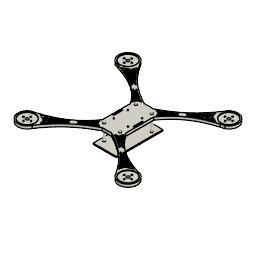
drone_frame_design (Autodesk Fusion 360 design; units mm, degrees)
part number: 2026-03-04-22-05-30-205
Autodesk Fusion 360 part; units mm, degrees
(part 1 of 3)
sketch "Sketch1" plane through (0, 0, 0) normal (0, 0, 1) x (1, 0, 0)
  line L0 (10, -45) -> (-10, -45)
  line L1 (-25, -30) -> (-25, 30)
  line L2 (-10, 45) -> (10, 45)
  line L3 (25, 30) -> (25, -30)
  line L4 (10, 45) -> (25, 30)
  line L5 (-25, 30) -> (-10, 45)
  line L6 (-10, -45) -> (-25, -30)
  line L7 (10, -45) -> (25, -30)
  circle A0 centre (108, 108) radius 20
  line L8 (0, 2.5) -> (0, 20)
  circle A1 centre (-108, 108) radius 20
  line L9 (20, 0) -> (2.5, 0)
  circle A2 centre (-108, -108) radius 20
  circle A3 centre (108, -108) radius 20
  line L10 (10, 45) -> (0, 45)
  spline S0 degree 5 poles (10, 45) (11.9791, 46.0284) (15.9034, 48.1188) (21.6887, 51.3552) (29.1964, 55.8754) (38.2146, 61.8908) (46.833, 68.3041) (55.0184, 75.1487) (62.7516, 82.4437) (70.0489, 90.1727) (76.9426, 98.3036) (82.1609, 105.1037) (85.9183, 110.3595) (88.3548, 113.9314) (89.5561, 115.7344) knots 0 0 0 0 0 0 0.1 0.2 0.3 0.4 0.5 0.6 0.7 0.8 0.9 1 1 1 1 1 1
  spline S1 degree 5 poles (25, 30) (26.2769, 31.7834) (28.8813, 35.2989) (32.9395, 40.4185) (38.6588, 46.9323) (46.356, 54.5193) (54.6474, 61.5042) (63.577, 67.8424) (73.161, 73.5176) (83.3647, 78.5649) (94.1376, 83.0355) (103.1721, 86.1903) (110.1669, 88.3346) (114.9258, 89.6671) (117.3292, 90.3092) knots 0 0 0 0 0 0 0.1 0.2 0.3 0.4 0.5 0.6 0.7 0.8 0.9 1 1 1 1 1 1
  spline S2 degree 5 poles (-10, 45) (-11.9791, 46.0284) (-15.9034, 48.1188) (-21.6887, 51.3552) (-29.1964, 55.8754) (-38.2146, 61.8908) (-46.833, 68.3041) (-55.0184, 75.1487) (-62.7516, 82.4437) (-70.0489, 90.1727) (-76.9426, 98.3036) (-82.1609, 105.1037) (-85.9183, 110.3595) (-88.3548, 113.9314) (-89.5561, 115.7344) knots 0 0 0 0 0 0 0.1 0.2 0.3 0.4 0.5 0.6 0.7 0.8 0.9 1 1 1 1 1 1
  line L11 (-0.5595, 39.5129) -> (20.5595, 50.4871)
  line L12 (83.0456, 105.9625) -> (96.0665, 125.5063)
  line L13 (0.5595, 39.5129) -> (-20.5595, 50.4871)
  line L14 (-83.0456, 105.9625) -> (-96.0665, 125.5063)
  spline S3 degree 5 poles (-25, 30) (-26.2769, 31.7834) (-28.8813, 35.2989) (-32.9395, 40.4185) (-38.6588, 46.9323) (-46.356, 54.5193) (-54.6474, 61.5042) (-63.577, 67.8424) (-73.161, 73.5176) (-83.3647, 78.5649) (-94.1376, 83.0355) (-103.1721, 86.1903) (-110.1669, 88.3346) (-114.9258, 89.6671) (-117.3292, 90.3092) knots 0 0 0 0 0 0 0.1 0.2 0.3 0.4 0.5 0.6 0.7 0.8 0.9 1 1 1 1 1 1
  line L15 (17.8241, 19.9779) -> (32.1759, 40.0221)
  line L16 (104.7277, 86.9428) -> (129.9307, 93.6755)
  line L17 (-17.8241, 19.9779) -> (-32.1759, 40.0221)
  line L18 (-104.7277, 86.9428) -> (-129.9307, 93.6755)
  spline S4 degree 5 poles (-25, -30) (-26.2769, -31.7834) (-28.8813, -35.2989) (-32.9395, -40.4185) (-38.6588, -46.9323) (-46.356, -54.5193) (-54.6474, -61.5042) (-63.577, -67.8424) (-73.161, -73.5176) (-83.3647, -78.5649) (-94.1376, -83.0355) (-103.1721, -86.1903) (-110.1669, -88.3346) (-114.9258, -89.6671) (-117.3292, -90.3092) knots 0 0 0 0 0 0 0.1 0.2 0.3 0.4 0.5 0.6 0.7 0.8 0.9 1 1 1 1 1 1
  line L19 (-17.8241, -19.9779) -> (-32.1759, -40.0221)
  line L20 (-104.7277, -86.9428) -> (-129.9307, -93.6755)
  spline S5 degree 5 poles (-10, -45) (-11.9791, -46.0284) (-15.9034, -48.1188) (-21.6887, -51.3552) (-29.1964, -55.8754) (-38.2146, -61.8908) (-46.833, -68.3041) (-55.0184, -75.1487) (-62.7516, -82.4437) (-70.0489, -90.1727) (-76.9426, -98.3036) (-82.1609, -105.1037) (-85.9183, -110.3595) (-88.3548, -113.9314) (-89.5561, -115.7344) knots 0 0 0 0 0 0 0.1 0.2 0.3 0.4 0.5 0.6 0.7 0.8 0.9 1 1 1 1 1 1
  line L21 (0.5595, -39.5129) -> (-20.5595, -50.4871)
  line L22 (-83.0456, -105.9625) -> (-96.0665, -125.5063)
  spline S6 degree 5 poles (10, -45) (11.9791, -46.0284) (15.9034, -48.1188) (21.6887, -51.3552) (29.1964, -55.8754) (38.2146, -61.8908) (46.833, -68.3041) (55.0184, -75.1487) (62.7516, -82.4437) (70.0489, -90.1727) (76.9426, -98.3036) (82.1609, -105.1037) (85.9183, -110.3595) (88.3548, -113.9314) (89.5561, -115.7344) knots 0 0 0 0 0 0 0.1 0.2 0.3 0.4 0.5 0.6 0.7 0.8 0.9 1 1 1 1 1 1
  line L23 (-0.5595, -39.5129) -> (20.5595, -50.4871)
  line L24 (83.0456, -105.9625) -> (96.0665, -125.5063)
  spline S7 degree 5 poles (25, -30) (26.2769, -31.7834) (28.8813, -35.2989) (32.9395, -40.4185) (38.6588, -46.9323) (46.356, -54.5193) (54.6474, -61.5042) (63.577, -67.8424) (73.161, -73.5176) (83.3647, -78.5649) (94.1376, -83.0355) (103.1721, -86.1903) (110.1669, -88.3346) (114.9258, -89.6671) (117.3292, -90.3092) knots 0 0 0 0 0 0 0.1 0.2 0.3 0.4 0.5 0.6 0.7 0.8 0.9 1 1 1 1 1 1
  line L25 (17.8241, -19.9779) -> (32.1759, -40.0221)
  line L26 (104.7277, -86.9428) -> (129.9307, -93.6755)
  line L27 (20, 0) -> (2.5, 0)
  line L28 (-128, 128) -> (-128, 108)
  line L29 (-128, -108) -> (-128, -128)
  line L30 (128, 128) -> (108, 128)
  line L31 (-108, 128) -> (-128, 128)
  line L32 (128, -128) -> (128, -108)
  line L33 (128, 108) -> (128, 128)
  line L34 (-128, -128) -> (-108, -128)
  line L35 (108, -128) -> (128, -128)
  point P0 (25, -45)
  point P1 (-25, -45)
  point P2 (-25, 45)
  point P3 (25, 45)
  point P4 (55.2098, 75.5318)
  point P5 (62.16, 66.6356)
  point P6 (-55.2098, 75.5318)
  point P7 (-62.16, 66.6356)
  point P8 (-62.16, -66.6356)
  point P9 (-55.2098, -75.5318)
  point P10 (55.2098, -75.5318)
  point P11 (62.16, -66.6356)
  dimension "d1" = 256
  dimension "d2" = 256
  dimension "d3" = 50
  dimension "d4" = 90
  dimension "d7" = 15
  dimension "d8" = 15
  dimension "d9" = 15
  dimension "d10" = 15
  dimension "d11" = 15
  dimension "d12" = 15
  dimension "d13" = 15
  dimension "d14" = 15
  dimension "d15" = 40
  constraint horizontal L30
  constraint perpendicular L28 L31
  constraint parallel L30 L35
  constraint parallel L28 L33
  constraint horizontal L0
  constraint perpendicular L0 L1
  constraint parallel L0 L2
  constraint parallel L1 L3
  constraint coincident P3 L2
  constraint coincident P3 L3
  constraint coincident P2 L1
  constraint coincident P2 L2
  constraint coincident P1 L0
  constraint coincident P1 L1
  constraint coincident P0 L0
  constraint coincident P0 L3
  constraint tangent A0 L30
  constraint tangent A0 L33
  constraint symmetric A0 L8 A1
  constraint symmetric A0 L9 A3
  constraint symmetric A1 L9 A2
  constraint midpoint L2 L10.end
  constraint symmetric L1 L3 L8
  constraint symmetric L0 L2 L9
  constraint coincident A0 S0.end
  constraint coincident A0 S1.end
  constraint midpoint L2.end L11
  constraint midpoint S0.end L12
  constraint midpoint L3.start L15
  constraint midpoint S1.end L16
  constraint symmetric L2.end L8 L2.start
  constraint symmetric L3.start L8 L1.end
  constraint symmetric L8 P4 P6
  constraint symmetric L8 S0.end S2.end
  constraint symmetric L8 P5 P7
  constraint symmetric L8 S1.end S3.end
  constraint symmetric L8 L11.start L13.start
  constraint symmetric L8 L11.end L13.end
  constraint symmetric L8 L12.start L14.start
  constraint symmetric L8 L12.end L14.end
  constraint symmetric L8 L15.start L17.start
  constraint symmetric L8 L15.end L17.end
  constraint symmetric L8 L16.start L18.start
  constraint symmetric L8 L16.end L18.end
  constraint symmetric L2.end L9 L0.start
  constraint symmetric L3.start L9 L3.end
  constraint symmetric L27.start L9 L9.start
  constraint symmetric L27.end L9 L9.end
  constraint symmetric L9 P4 P10
  constraint symmetric L9 S0.end S6.end
  constraint symmetric L9 P5 P11
  constraint symmetric L9 S1.end S7.end
  constraint symmetric L9 L2.start L0.end
  constraint symmetric L9 P6 P9
  constraint symmetric L9 S2.end S5.end
  constraint symmetric L9 L11.start L23.start
  constraint symmetric L9 L11.end L23.end
  constraint symmetric L9 L12.start L24.start
  constraint symmetric L9 L12.end L24.end
  constraint symmetric L9 L13.start L21.start
  constraint symmetric L9 L13.end L21.end
  constraint symmetric L9 L14.start L22.start
  constraint symmetric L9 L14.end L22.end
  constraint symmetric L9 L1.end L1.start
  constraint symmetric L9 P7 P8
  constraint symmetric L9 S3.end S4.end
  constraint symmetric L9 L15.start L25.start
  constraint symmetric L9 L15.end L25.end
  constraint symmetric L9 L16.start L26.start
  constraint symmetric L9 L16.end L26.end
  constraint symmetric L9 L17.start L19.start
  constraint symmetric L9 L17.end L19.end
  constraint symmetric L9 L18.start L20.start
  constraint symmetric L9 L18.end L20.end
  constraint coincident A1 L28.end
  constraint coincident A2 L29.start
  constraint collinear L28 L29
  constraint coincident A0 L30.end
  constraint coincident A1 L31.start
  constraint collinear L30 L31
  constraint coincident A3 L32.end
  constraint coincident A0 L33.start
  constraint collinear L32 L33
  constraint coincident A2 L34.end
  constraint coincident A3 L35.start
  constraint collinear L34 L35
  measures "d1" distance of L29.end L32.start
  measures "d2" distance of L28.start L29.end
  measures "d3" distance of P2 P3
  measures "d4" distance of P1 P2
  measures "d7" distance of P3 L2.end L29.end
  measures "d8" distance of P3 L3.start L29.end
  measures "d9" distance of P2 L1.end
  measures "d10" distance of P2 L2.start
  measures "d11" distance of P1 L0.end
  measures "d12" distance of P1 L1.start
  measures "d13" distance of P0 L0.start
  measures "d14" distance of P0 L3.end
  measures "d15" diameter of A0
sketch "Sketch3" plane through (0, 0, 0) normal (0, 0, 1) x (1, 0, 0)
extrude "Extrude1" add sketch "Sketch1" along normal blind 6 contours L1 L3 L4 L5 L6 L7 L11 L13 L21 L23 | L0 L21 L23 | L2 L10 L11 L13 makes body 1
extrude "Extrude2" add sketch "Sketch1" along normal blind 6 contours L7 A3 S6 S7 | L6 A2 S4 S5 | L4 A0 S0 S1 | L5 A1 S2 S3 bodies 1
sketch "Sketch4" plane through (0, 0, 6) normal (0, 0, 1) x (-1, 0, 0)
  spline S0 degree 5 poles (-10, 45) (-11.9791, 46.0284) (-15.9034, 48.1188) (-21.6887, 51.3552) (-29.1964, 55.8754) (-38.2146, 61.8908) (-46.833, 68.3041) (-55.0184, 75.1487) (-62.7516, 82.4437) (-70.0489, 90.1727) (-76.9426, 98.3036) (-82.1609, 105.1037) (-85.9183, 110.3595) (-88.3548, 113.9314) (-89.5561, 115.7344) knots 0 0 0 0 0 0 0.1 0.2 0.3 0.4 0.5 0.6 0.7 0.8 0.9 1 1 1 1 1 1
  arc A0 (-109.3801, 88.0477) -> (-89.5561, 115.7344) centre (-108, 108) ccw
  spline S1 degree 5 poles (-109.3801, 88.0477) (-108.6093, 87.8146) (-105.5101, 86.8635) (-100.1552, 85.1208) (-92.6931, 82.436) (-83.3647, 78.5649) (-73.161, 73.5176) (-63.577, 67.8424) (-54.6474, 61.5042) (-46.356, 54.5193) (-38.6588, 46.9323) (-32.9395, 40.4185) (-28.8813, 35.2989) (-26.2769, 31.7834) (-25, 30) knots -0.932954 -0.932954 -0.932954 -0.932954 -0.932954 -0.932954 -0.9 -0.8 -0.7 -0.6 -0.5 -0.4 -0.3 -0.2 -0.1 0 0 0 0 0 0
  line L0 (-10, 45) -> (-25, 30)
  line L1 (-10, -45) -> (10, -45)
  spline S2 degree 5 poles (10, -45) (11.9791, -46.0284) (15.9034, -48.1188) (21.6887, -51.3552) (29.1964, -55.8754) (38.2146, -61.8908) (46.833, -68.3041) (55.0184, -75.1487) (62.7516, -82.4437) (70.0489, -90.1727) (76.9426, -98.3036) (82.1609, -105.1037) (85.9183, -110.3595) (88.3548, -113.9314) (89.5561, -115.7344) knots 0 0 0 0 0 0 0.1 0.2 0.3 0.4 0.5 0.6 0.7 0.8 0.9 1 1 1 1 1 1
  arc A1 (109.3801, -88.0477) -> (89.5561, -115.7344) centre (108, -108) ccw
  spline S3 degree 5 poles (109.3801, -88.0477) (108.6093, -87.8146) (105.5101, -86.8635) (100.1552, -85.1208) (92.6931, -82.436) (83.3647, -78.5649) (73.161, -73.5176) (63.577, -67.8424) (54.6474, -61.5042) (46.356, -54.5193) (38.6588, -46.9323) (32.9395, -40.4185) (28.8813, -35.2989) (26.2769, -31.7834) (25, -30) knots -0.932954 -0.932954 -0.932954 -0.932954 -0.932954 -0.932954 -0.9 -0.8 -0.7 -0.6 -0.5 -0.4 -0.3 -0.2 -0.1 0 0 0 0 0 0
  line L2 (25, -30) -> (25, 30)
  spline S4 degree 5 poles (25, 30) (26.2769, 31.7834) (28.8813, 35.2989) (32.9395, 40.4185) (38.6588, 46.9323) (46.356, 54.5193) (54.6474, 61.5042) (63.577, 67.8424) (73.161, 73.5176) (83.3647, 78.5649) (92.6931, 82.436) (100.1552, 85.1208) (105.5101, 86.8635) (108.6093, 87.8146) (109.3801, 88.0477) knots 0 0 0 0 0 0 0.1 0.2 0.3 0.4 0.5 0.6 0.7 0.8 0.9 0.932954 0.932954 0.932954 0.932954 0.932954 0.932954
  arc A2 (89.5561, 115.7344) -> (109.3801, 88.0477) centre (108, 108) ccw
  spline S5 degree 5 poles (89.5561, 115.7344) (88.3548, 113.9314) (85.9183, 110.3595) (82.1609, 105.1037) (76.9426, 98.3036) (70.0489, 90.1727) (62.7516, 82.4437) (55.0184, 75.1487) (46.833, 68.3041) (38.2146, 61.8908) (29.1964, 55.8754) (21.6887, 51.3552) (15.9034, 48.1188) (11.9791, 46.0284) (10, 45) knots -1 -1 -1 -1 -1 -1 -0.9 -0.8 -0.7 -0.6 -0.5 -0.4 -0.3 -0.2 -0.1 0 0 0 0 0 0
  line L3 (10, 45) -> (-10, 45)
  line L4 (-25, 30) -> (-25, -30)
  spline S6 degree 5 poles (-25, -30) (-26.2769, -31.7834) (-28.8813, -35.2989) (-32.9395, -40.4185) (-38.6588, -46.9323) (-46.356, -54.5193) (-54.6474, -61.5042) (-63.577, -67.8424) (-73.161, -73.5176) (-83.3647, -78.5649) (-92.6931, -82.436) (-100.1552, -85.1208) (-105.5101, -86.8635) (-108.6093, -87.8146) (-109.3801, -88.0477) knots 0 0 0 0 0 0 0.1 0.2 0.3 0.4 0.5 0.6 0.7 0.8 0.9 0.932954 0.932954 0.932954 0.932954 0.932954 0.932954
  arc A3 (-89.5561, -115.7344) -> (-109.3801, -88.0477) centre (-108, -108) ccw
  spline S7 degree 5 poles (-89.5561, -115.7344) (-88.3548, -113.9314) (-85.9183, -110.3595) (-82.1609, -105.1037) (-76.9426, -98.3036) (-70.0489, -90.1727) (-62.7516, -82.4437) (-55.0184, -75.1487) (-46.833, -68.3041) (-38.2146, -61.8908) (-29.1964, -55.8754) (-21.6887, -51.3552) (-15.9034, -48.1188) (-11.9791, -46.0284) (-10, -45) knots -1 -1 -1 -1 -1 -1 -0.9 -0.8 -0.7 -0.6 -0.5 -0.4 -0.3 -0.2 -0.1 0 0 0 0 0 0
sketch "Sketch5" plane through (0, 0, 6) normal (0, 0, 1) x (-1, 0, 0)
  spline S0 degree 5 poles (-25, -30) (-26.2769, -31.7834) (-28.8813, -35.2989) (-32.9395, -40.4185) (-38.6588, -46.9323) (-46.356, -54.5193) (-54.6474, -61.5042) (-63.577, -67.8424) (-73.161, -73.5176) (-83.3647, -78.5649) (-92.6931, -82.436) (-100.1552, -85.1208) (-105.5101, -86.8635) (-108.6093, -87.8146) (-109.3801, -88.0477) knots 0 0 0 0 0 0 0.1 0.2 0.3 0.4 0.5 0.6 0.7 0.8 0.9 0.932954 0.932954 0.932954 0.932954 0.932954 0.932954
  arc A0 (-89.5561, -115.7344) -> (-109.3801, -88.0477) centre (-108, -108) ccw
  spline S1 degree 5 poles (-89.5561, -115.7344) (-88.3548, -113.9314) (-85.9183, -110.3595) (-82.1609, -105.1037) (-76.9426, -98.3036) (-70.0489, -90.1727) (-62.7516, -82.4437) (-55.0184, -75.1487) (-46.833, -68.3041) (-38.2146, -61.8908) (-29.1964, -55.8754) (-21.6887, -51.3552) (-15.9034, -48.1188) (-11.9791, -46.0284) (-10, -45) knots -1 -1 -1 -1 -1 -1 -0.9 -0.8 -0.7 -0.6 -0.5 -0.4 -0.3 -0.2 -0.1 0 0 0 0 0 0
  line L0 (-16.6491, -44.0078) -> (-24.5394, -36.1175)
  line L1 (-16.6491, -44.0078) -> (-15.7266, -44.9303)
  line L2 (-24.5394, -36.1175) -> (-26.1093, -34.5476)
  spline S2 degree 3 poles (-86.4629, -107.5181) (-77.6632, -95.0692) (-67.8257, -83.6168) (-56.6007, -73.5039) (-44.7534, -62.8301) (-31.3991, -53.6699) (-16.9588, -45.6135) (-16.549, -45.3849) (-16.1382, -45.1571) (-15.7266, -44.9303) knots -0.921557 -0.921557 -0.921557 -0.921557 -0.5 -0.5 -0.5 -0.055069 -0.055069 -0.055069 -0.042441 -0.042441 -0.042441 -0.042441
  spline S3 degree 3 poles (-26.1093, -34.5476) (-33.7424, -44.66) (-42.377, -53.7768) (-52.2721, -61.6437) (-60.5587, -68.2317) (-69.767, -73.8901) (-79.7914, -78.6767) (-86.5715, -81.9141) (-93.7109, -84.7689) (-101.1598, -87.3016) knots 0.039267 0.039267 0.039267 0.039267 0.383484 0.383484 0.383484 0.671746 0.671746 0.671746 0.86671 0.86671 0.86671 0.86671
  circle A1 centre (-108, -108) radius 20
  line L3 (-21.0824, -39.4285) -> (-91.6554, -96.5652)
  line L4 (-19.9851, -40.7292) -> (-90.7737, -97.8385)
  line L5 (-15.7266, -44.9303) -> (-22.1293, -42.4591)
  line L6 (-22.1293, -42.4591) -> (-21.2525, -48.0608)
  line L7 (-23.5672, -43.6191) -> (-22.7358, -48.9312)
  line L8 (-18.5197, -42.1372) -> (-20.6913, -41.299)
  line L9 (-22.7358, -48.9312) -> (-27.7829, -47.0202)
  line L10 (-6.9172, 6.1796) -> (-6.9171, 6.1796)
  line L11 (-6.9171, 6.1796) -> (-6.9172, 6.1796)
  line L12 (0, 0) -> (0, 45)
  line L13 (0, 0) -> (0, -45)
  line L14 (10, -45) -> (-10, -45)
  circle A2 centre (15.25, -15.25) radius 1.5
  circle A3 centre (-15.25, -15.25) radius 1.5
  line L15 (-6.9171, 6.1796) -> (-6.9172, 6.1796)
  line L16 (0, 0) -> (0, 45)
  line L17 (-25, -30) -> (-25, 30)
  line L18 (25, 30) -> (25, -30)
  line L19 (25, 0) -> (-25, 0)
  circle A4 centre (15.25, 15.25) radius 1.5
  circle A5 centre (-15.25, 15.25) radius 1.5
  line L20 (23.3348, 0) -> (23.3348, -9)
  line L21 (23.3348, 0) -> (23.3348, 9)
  line L22 (20.8348, 0) -> (20.8348, -9)
  line L23 (20.8348, 0) -> (20.8348, 9)
  line L24 (22.3348, -10) -> (21.8348, -10)
  line L25 (22.3348, 10) -> (21.8348, 10)
  arc A6 (20.8348, -9) -> (21.8348, -10) centre (21.8348, -9) ccw
  arc A7 (22.3348, -10) -> (23.3348, -9) centre (22.3348, -9) ccw
  arc A8 (23.3348, 9) -> (22.3348, 10) centre (22.3348, 9) ccw
  arc A9 (21.8348, 10) -> (20.8348, 9) centre (21.8348, 9) ccw
  line L26 (-20.8348, 0) -> (-20.8348, -9)
  line L27 (-23.3348, 0) -> (-23.3348, -9)
  arc A10 (-23.3348, -9) -> (-22.3348, -10) centre (-22.3348, -9) ccw
  line L28 (-22.3348, -10) -> (-21.8348, -10)
  arc A11 (-21.8348, -10) -> (-20.8348, -9) centre (-21.8348, -9) ccw
  line L29 (-20.8348, 0) -> (-20.8348, 9)
  arc A12 (-20.8348, 9) -> (-21.8348, 10) centre (-21.8348, 9) ccw
  line L30 (-23.3348, 0) -> (-23.3348, 9)
  arc A13 (-22.3348, 10) -> (-23.3348, 9) centre (-22.3348, 9) ccw
  line L31 (-22.3348, 10) -> (-21.8348, 10)
  line L32 (-21.9883, -43.3599) -> (-21.2525, -48.0608)
  line L33 (-24.4898, -49.9779) -> (-28.3781, -48.5056)
  line L34 (-28.3781, -48.5056) -> (-29.2262, -48.1845)
  line L35 (-29.2262, -48.1845) -> (-29.2262, -52.9038)
  line L36 (-23.9305, -48.4789) -> (-27.8043, -47.0121)
  line L37 (-30.8262, -49.4754) -> (-30.8262, -52.9129)
  line L38 (-30.8262, -52.9129) -> (-30.8262, -53.9269)
  line L39 (-30.8262, -53.9269) -> (-35.0824, -52.9091)
  line L40 (-53.3931, -70.682) -> (-58.101, -66.0186)
  line L41 (-29.2262, -49.4693) -> (-29.2262, -52.9129)
  line L42 (-32.6725, -55.1305) -> (-35.4701, -54.4615)
  line L43 (-35.4701, -54.4615) -> (-36.6553, -54.1781)
  line L44 (-36.6553, -54.1781) -> (-36.873, -57.9658)
  line L45 (-32.3111, -53.5718) -> (-35.0977, -52.9055)
  line L46 (-38.3359, -55.5339) -> (-38.471, -57.8848)
  line L47 (-38.471, -57.8848) -> (-38.5427, -59.1325)
  line L48 (-38.5427, -59.1325) -> (-42.6724, -59.0324)
  line L49 (-36.7393, -55.6397) -> (-36.8736, -57.9769)
  line L50 (-40.7069, -60.6805) -> (-42.7105, -60.6319)
  line L51 (-42.7105, -60.6319) -> (-44.5984, -60.5862)
  line L52 (-44.5984, -60.5862) -> (-45.0116, -63.8871)
  line L53 (-45.0116, -63.8871) -> (-49.5335, -59.4079)
  line L54 (-53.3931, -70.682) -> (-57.6141, -71.0867)
  line L55 (-57.6141, -71.0867) -> (-58.1695, -74.9342)
  line L56 (-59.4437, -72.5628) -> (-59.7672, -74.8031)
  line L57 (-59.7672, -74.8031) -> (-60.0386, -76.6835)
  line L58 (-60.0386, -76.6835) -> (-64.4078, -76.5676)
  line L59 (-57.8815, -72.939) -> (-58.1478, -74.7839)
  line L60 (-61.6594, -78.2411) -> (-64.4912, -78.166)
  line L61 (-64.4912, -78.166) -> (-66.3286, -78.1172)
  line L62 (-66.3286, -78.1172) -> (-66.0088, -82.615)
  line L63 (-61.718, -76.639) -> (-64.4987, -76.5652)
  line L64 (-67.8456, -79.3411) -> (-67.6012, -82.7793)
  line L65 (-67.6012, -82.7793) -> (-67.5013, -84.1835)
  line L66 (-67.5013, -84.1835) -> (-72.3151, -82.9469)
  line L67 (-66.2418, -79.3387) -> (-66.006, -82.6541)
  line L68 (-68.7436, -85.5164) -> (-72.6899, -84.5025)
  line L69 (-72.6899, -84.5025) -> (-73.8681, -84.1998)
  line L70 (-73.8681, -84.1998) -> (-72.3108, -89.4858)
  line L71 (-68.3889, -83.9555) -> (-72.2959, -82.9518)
  line L72 (-75.2158, -85.2871) -> (-73.8403, -89.9558)
  line L73 (-73.8403, -89.9558) -> (-73.5557, -90.9221)
  line L74 (-73.5557, -90.9221) -> (-79.0459, -88.377)
  line L75 (-73.6551, -84.9229) -> (-72.3584, -89.3243)
  line L76 (-74.6324, -92.1865) -> (-79.6597, -89.856)
  line L77 (-79.6597, -89.856) -> (-80.4342, -89.497)
  line L78 (-80.4342, -89.497) -> (-77.8281, -96.0622)
  line L79 (-73.975, -90.7277) -> (-78.9919, -88.4021)
  line L80 (-81.7381, -90.5489) -> (-79.314, -96.6555)
  line L81 (-79.314, -96.6555) -> (-78.9776, -97.5027)
  line L82 (-78.9776, -97.5027) -> (-85.6123, -93.6745)
  line L83 (-80.2171, -90.0439) -> (-77.908, -95.8607)
  line L84 (-79.9758, -98.774) -> (-86.334, -95.1053)
  line L85 (-86.334, -95.1053) -> (-86.9472, -94.7515)
  line L86 (-79.1831, -97.3842) -> (-85.5398, -93.7163)
  line L87 (-84.24, -103.2596) -> (-83.881, -103.9354)
  line L88 (-86.4629, -107.5181) -> (-88.083, -109.8203)
  line L89 (-84.9411, -105.1338) -> (-89.1017, -101.4536)
  line L90 (-23.1969, -41.1404) -> (-26.1093, -34.5476)
  line L91 (-23.1969, -41.1404) -> (-29.7792, -39.2354)
  line L92 (-21.9085, -40.0973) -> (-22.9759, -37.6809)
  line L93 (-24.7124, -42.3674) -> (-30.224, -40.7724)
  line L94 (-30.224, -40.7724) -> (-30.8842, -40.5813)
  line L95 (-30.8842, -40.5813) -> (-29.0347, -45.8668)
  line L96 (-32.0809, -42.0059) -> (-30.545, -46.3953)
  line L97 (-30.545, -46.3953) -> (-30.3557, -46.9362)
  line L98 (-30.3557, -46.9362) -> (-35.1263, -45.4835)
  line L99 (-31.8569, -48.1516) -> (-35.5924, -47.0141)
  line L100 (-35.5924, -47.0141) -> (-36.3212, -46.7922)
  line L101 (-36.3212, -46.7922) -> (-36.3212, -51.766)
  line L102 (-37.9212, -48.4975) -> (-37.9212, -51.766)
  line L103 (-37.9212, -51.766) -> (-37.9212, -53.0614)
  line L104 (-37.9212, -53.0614) -> (-41.7959, -52.4137)
  line L105 (-39.5819, -54.4059) -> (-42.0597, -53.9918)
  line L106 (-42.0597, -53.9918) -> (-43.2354, -53.7952)
  line L107 (-43.2354, -53.7952) -> (-43.6369, -57.6889)
  line L108 (-45.0146, -55.4505) -> (-45.2285, -57.5248)
  line L109 (-45.2285, -57.5248) -> (-45.3919, -59.1098)
  line L110 (-45.3919, -59.1098) -> (-49.5335, -59.4079)
  line L111 (-47.5667, -60.8705) -> (-48.0238, -60.9034)
  line L112 (-46.392, -62.0332) -> (-46.4462, -62.4661)
  line L113 (-58.101, -66.0186) -> (-58.8192, -69.9806)
  line L114 (-58.8192, -69.9806) -> (-63.64, -69.7432)
  line L115 (-60.6844, -71.4907) -> (-63.7187, -71.3413)
  line L116 (-63.7187, -71.3413) -> (-66.0187, -71.228)
  line L117 (-66.0187, -71.228) -> (-65.6021, -75.4722)
  line L118 (-67.5366, -72.1422) -> (-67.1945, -75.6285)
  line L119 (-67.1945, -75.6285) -> (-67.0915, -76.678)
  line L120 (-67.0915, -76.678) -> (-73.3235, -75.4057)
  line L121 (-68.7023, -77.9821) -> (-73.6436, -76.9733)
  line L122 (-73.6436, -76.9733) -> (-75.564, -76.5813)
  line L123 (-75.564, -76.5813) -> (-73.4538, -81.829)
  line L124 (-76.996, -77.3086) -> (-74.9383, -82.4259)
  line L125 (-74.9383, -82.4259) -> (-74.7548, -82.8823)
  line L126 (-74.7548, -82.8823) -> (-82.0425, -79.7315)
  line L127 (-76.1584, -84.0186) -> (-82.6775, -81.2002)
  line L128 (-82.6775, -81.2002) -> (-84.0126, -80.6229)
  line L129 (-84.0126, -80.6229) -> (-80.1679, -87.2648)
  line L130 (-85.3974, -81.4245) -> (-81.5527, -88.0664)
  line L131 (-81.5527, -88.0664) -> (-81.4267, -88.284)
  line L132 (-85.3974, -81.4245) -> (-85.4862, -81.271)
  line L133 (-81.4267, -88.284) -> (-90.517, -83.3708)
  line L134 (-82.7739, -89.3746) -> (-91.2777, -84.7783)
  line L135 (-91.2777, -84.7783) -> (-92.4617, -84.1384)
  line L136 (-92.4617, -84.1384) -> (-86.7336, -92.5805)
  line L137 (-93.7857, -85.0368) -> (-87.9816, -93.5909)
  line L138 (-93.7857, -85.0368) -> (-93.9955, -84.7275)
  line L139 (-101.1598, -87.3016) -> (-104.0335, -88.3973)
  line L140 (-87.9816, -93.5909) -> (-100.8677, -87.202)
  line L141 (-89.3497, -94.6985) -> (-101.5784, -88.6355)
  line L142 (-101.5784, -88.6355) -> (-102.9173, -87.9717)
  line L143 (79.9758, -98.774) -> (86.334, -95.1053)
  line L144 (59.4437, -72.5628) -> (59.7672, -74.8031)
  line L145 (24.5394, -36.1175) -> (26.1093, -34.5476)
  line L146 (23.1969, -41.1404) -> (29.7792, -39.2354)
  line L147 (27.8043, -47.0121) -> (29.0347, -45.8668)
  line L148 (23.9305, -48.4789) -> (27.8043, -47.0121)
  line L149 (29.2262, -49.4693) -> (29.2262, -52.9129)
  line L150 (21.9883, -43.3599) -> (21.2525, -48.0608)
  line L151 (36.7393, -55.6397) -> (36.8736, -57.9769)
  line L152 (45.2285, -57.5248) -> (45.3919, -59.1098)
  line L153 (35.5924, -47.0141) -> (36.3212, -46.7922)
  line L154 (36.6553, -54.1781) -> (36.873, -57.9658)
  line L155 (40.7069, -60.6805) -> (42.7105, -60.6319)
  line L156 (43.2354, -53.7952) -> (43.6369, -57.6889)
  line L157 (32.3111, -53.5718) -> (35.0977, -52.9055)
  line L158 (36.3212, -46.7922) -> (36.3212, -51.766)
  line L159 (16.6491, -44.0078) -> (15.7266, -44.9303)
  line L160 (29.2262, -48.1845) -> (29.2262, -52.9038)
  line L161 (30.8262, -49.4754) -> (30.8262, -52.9129)
  line L162 (35.4701, -54.4615) -> (36.6553, -54.1781)
  line L163 (42.7105, -60.6319) -> (44.5984, -60.5862)
  line L164 (16.6491, -44.0078) -> (24.5394, -36.1175)
  line L165 (38.471, -57.8848) -> (38.5427, -59.1325)
  line L166 (18.5197, -42.1372) -> (20.6913, -41.299)
  line L167 (42.0597, -53.9918) -> (43.2354, -53.7952)
  line L168 (22.1293, -42.4591) -> (23.1969, -41.1404)
  line L169 (80.4342, -89.497) -> (77.8281, -96.0622)
  line L170 (79.6597, -89.856) -> (80.4342, -89.497)
  line L171 (67.8456, -79.3411) -> (67.6012, -82.7793)
  line L172 (68.7436, -85.5164) -> (72.6899, -84.5025)
  line L173 (73.975, -90.7277) -> (78.9919, -88.4021)
  line L174 (73.5557, -90.9221) -> (79.0459, -88.377)
  line L175 (73.8403, -89.9558) -> (73.5557, -90.9221)
  line L176 (68.3889, -83.9555) -> (72.2959, -82.9518)
  line L177 (74.6324, -92.1865) -> (79.6597, -89.856)
  line L178 (74.9383, -82.4259) -> (74.7548, -82.8823)
  line L179 (66.2418, -79.3387) -> (66.006, -82.6541)
  line L180 (75.2158, -85.2871) -> (73.8403, -89.9558)
  line L181 (66.0187, -71.228) -> (65.6021, -75.4722)
  line L182 (67.5366, -72.1422) -> (67.1945, -75.6285)
  line L183 (64.4987, -76.5652) -> (65.6021, -75.4722)
  line L184 (64.4912, -78.166) -> (66.3286, -78.1172)
  line L185 (61.6594, -78.2411) -> (64.4912, -78.166)
  line L186 (81.7381, -90.5489) -> (79.314, -96.6555)
  line L187 (74.7548, -82.8823) -> (82.0425, -79.7315)
  line L188 (58.8192, -69.9806) -> (63.64, -69.7432)
  line L189 (63.7187, -71.3413) -> (66.0187, -71.228)
  line L190 (59.7672, -74.8031) -> (60.0386, -76.6835)
  line L191 (79.1831, -97.3842) -> (85.5398, -93.7163)
  line L192 (84.0126, -80.6229) -> (80.1679, -87.2648)
  line L193 (73.6436, -76.9733) -> (75.564, -76.5813)
  line L194 (60.0386, -76.6835) -> (64.4078, -76.5676)
  line L195 (46.392, -62.0332) -> (46.4462, -62.4661)
  line L196 (45.3919, -59.1098) -> (49.5335, -59.4079)
  line L197 (45.0146, -55.4505) -> (45.2285, -57.5248)
  line L198 (44.5984, -60.5862) -> (45.0116, -63.8871)
  line L199 (38.5427, -59.1325) -> (42.6724, -59.0324)
  line L200 (45.0116, -63.8871) -> (49.5335, -59.4079)
  line L201 (21.0824, -39.4285) -> (91.6554, -96.5652)
  line L202 (89.3497, -94.6985) -> (101.5784, -88.6355)
  line L203 (85.3974, -81.4245) -> (85.4862, -81.271)
  line L204 (81.4267, -88.284) -> (90.517, -83.3708)
  spline S4 degree 3 poles (26.1093, -34.5476) (33.7424, -44.66) (42.377, -53.7768) (52.2721, -61.6437) (60.5587, -68.2317) (69.767, -73.8901) (79.7914, -78.6767) (86.5715, -81.9141) (93.7109, -84.7689) (101.1598, -87.3016) knots 0.039267 0.039267 0.039267 0.039267 0.383484 0.383484 0.383484 0.671746 0.671746 0.671746 0.86671 0.86671 0.86671 0.86671
  line L205 (82.6775, -81.2002) -> (84.0126, -80.6229)
  line L206 (84.9411, -105.1338) -> (89.1017, -101.4536)
  line L207 (92.4617, -84.1384) -> (86.7336, -92.5805)
  spline S5 degree 3 poles (86.4629, -107.5181) (77.6632, -95.0692) (67.8257, -83.6168) (56.6007, -73.5039) (44.7534, -62.8301) (31.3991, -53.6699) (16.9588, -45.6135) (16.549, -45.3849) (16.1382, -45.1571) (15.7266, -44.9303) knots -0.921557 -0.921557 -0.921557 -0.921557 -0.5 -0.5 -0.5 -0.055069 -0.055069 -0.055069 -0.042441 -0.042441 -0.042441 -0.042441
  line L208 (91.2777, -84.7783) -> (92.4617, -84.1384)
  line L209 (60.6844, -71.4907) -> (63.7187, -71.3413)
  line L210 (67.0915, -76.678) -> (73.3235, -75.4057)
  line L211 (53.3931, -70.682) -> (57.6141, -71.0867)
  line L212 (53.3931, -70.682) -> (58.101, -66.0186)
  line L213 (57.8815, -72.939) -> (58.1478, -74.7839)
  line L214 (68.7023, -77.9821) -> (73.6436, -76.9733)
  line L215 (37.9212, -51.766) -> (37.9212, -53.0614)
  line L216 (47.5667, -60.8705) -> (48.0238, -60.9034)
  line L217 (37.9212, -53.0614) -> (41.7959, -52.4137)
  line L218 (32.6725, -55.1305) -> (35.4701, -54.4615)
  line L219 (37.9212, -48.4975) -> (37.9212, -51.766)
  line L220 (39.5819, -54.4059) -> (42.0597, -53.9918)
  line L221 (87.9816, -93.5909) -> (100.8677, -87.202)
  line L222 (83.881, -103.9354) -> (90.7737, -97.8385)
  line L223 (101.1598, -87.3016) -> (104.0335, -88.3973)
  line L224 (85.3974, -81.4245) -> (81.5527, -88.0664)
  line L225 (84.24, -103.2596) -> (83.881, -103.9354)
  line L226 (101.5784, -88.6355) -> (102.9173, -87.9717)
  arc A14 (109.3801, -88.0477) -> (89.5561, -115.7344) centre (108, -108) ccw
  line L227 (93.7857, -85.0368) -> (93.9955, -84.7275)
  line L228 (86.4629, -107.5181) -> (88.083, -109.8203)
  line L229 (93.7857, -85.0368) -> (87.9816, -93.5909)
  line L230 (81.5527, -88.0664) -> (81.4267, -88.284)
  line L231 (86.334, -95.1053) -> (86.9472, -94.7515)
  line L232 (82.7739, -89.3746) -> (91.2777, -84.7783)
  line L233 (67.5013, -84.1835) -> (72.3151, -82.9469)
  line L234 (66.3286, -78.1172) -> (66.0088, -82.615)
  line L235 (67.6012, -82.7793) -> (67.5013, -84.1835)
  line L236 (72.6899, -84.5025) -> (73.8681, -84.1998)
  line L237 (80.2171, -90.0439) -> (77.908, -95.8607)
  spline S6 degree 5 poles (89.5561, -115.7344) (88.3548, -113.9314) (85.9183, -110.3595) (82.1609, -105.1037) (76.9426, -98.3036) (70.0489, -90.1727) (62.7516, -82.4437) (55.0184, -75.1487) (46.833, -68.3041) (38.2146, -61.8908) (29.1964, -55.8754) (21.6887, -51.3552) (15.9034, -48.1188) (11.9791, -46.0284) (10, -45) knots -1 -1 -1 -1 -1 -1 -0.9 -0.8 -0.7 -0.6 -0.5 -0.4 -0.3 -0.2 -0.1 0 0 0 0 0 0
  line L238 (73.6551, -84.9229) -> (72.3584, -89.3243)
  line L239 (76.996, -77.3086) -> (74.9383, -82.4259)
  line L240 (73.8681, -84.1998) -> (72.3108, -89.4858)
  line L241 (79.314, -96.6555) -> (78.9776, -97.5027)
  line L242 (75.564, -76.5813) -> (73.4538, -81.829)
  line L243 (76.1584, -84.0186) -> (82.6775, -81.2002)
  line L244 (78.9776, -97.5027) -> (85.6123, -93.6745)
  line L245 (30.8262, -53.9269) -> (35.0824, -52.9091)
  line L246 (30.3557, -46.9362) -> (35.1263, -45.4835)
  line L247 (31.8569, -48.1516) -> (35.5924, -47.0141)
  line L248 (32.0809, -42.0059) -> (30.545, -46.3953)
  line L249 (38.3359, -55.5339) -> (38.471, -57.8848)
  line L250 (57.6141, -71.0867) -> (58.1695, -74.9342)
  line L251 (61.718, -76.639) -> (64.4987, -76.5652)
  line L252 (58.101, -66.0186) -> (58.8192, -69.9806)
  line L253 (67.1945, -75.6285) -> (67.0915, -76.678)
  line L254 (19.9851, -40.7292) -> (90.7737, -97.8385)
  line L255 (30.8842, -40.5813) -> (29.0347, -45.8668)
  line L256 (30.224, -40.7724) -> (30.8842, -40.5813)
  line L257 (30.545, -46.3953) -> (30.3557, -46.9362)
  line L258 (30.8262, -52.9129) -> (30.8262, -53.9269)
  line L259 (15.7266, -44.9303) -> (22.1293, -42.4591)
  line L260 (22.7358, -48.9312) -> (27.7829, -47.0202)
  line L261 (22.1293, -42.4591) -> (21.2525, -48.0608)
  line L262 (23.5672, -43.6191) -> (22.7358, -48.9312)
  line L263 (24.7124, -42.3674) -> (30.224, -40.7724)
  line L264 (21.9085, -40.0973) -> (22.9759, -37.6809)
  line L265 (23.1969, -41.1404) -> (26.1093, -34.5476)
  line L266 (28.3781, -48.5056) -> (29.2262, -48.1845)
  line L267 (24.4898, -49.9779) -> (28.3781, -48.5056)
  line L268 (23.1969, 41.1404) -> (26.1093, 34.5476)
  line L269 (16.6491, 44.0078) -> (15.7266, 44.9303)
  line L270 (23.9305, 48.4789) -> (27.8043, 47.0121)
  line L271 (22.1293, 42.4591) -> (23.1969, 41.1404)
  line L272 (10, 45) -> (-10, 45)
  line L273 (21.9085, 40.0973) -> (22.9759, 37.6809)
  line L274 (18.5197, 42.1372) -> (20.6913, 41.299)
  line L275 (38.471, 57.8848) -> (38.5427, 59.1325)
  line L276 (24.4898, 49.9779) -> (28.3781, 48.5056)
  line L277 (23.1969, 41.1404) -> (29.7792, 39.2354)
  line L278 (36.6553, 54.1781) -> (36.873, 57.9658)
  line L279 (36.3212, 46.7922) -> (36.3212, 51.766)
  line L280 (30.3557, 46.9362) -> (35.1263, 45.4835)
  line L281 (30.545, 46.3953) -> (30.3557, 46.9362)
  line L282 (30.224, 40.7724) -> (30.8842, 40.5813)
  line L283 (27.8043, 47.0121) -> (29.0347, 45.8668)
  line L284 (30.8262, 53.9269) -> (35.0824, 52.9091)
  line L285 (28.3781, 48.5056) -> (29.2262, 48.1845)
  line L286 (24.7124, 42.3674) -> (30.224, 40.7724)
  line L287 (38.3359, 55.5339) -> (38.471, 57.8848)
  line L288 (44.5984, 60.5862) -> (45.0116, 63.8871)
  line L289 (37.9212, 48.4975) -> (37.9212, 51.766)
  line L290 (38.5427, 59.1325) -> (42.6724, 59.0324)
  line L291 (47.5667, 60.8705) -> (48.0238, 60.9034)
  line L292 (30.8842, 40.5813) -> (29.0347, 45.8668)
  line L293 (42.0597, 53.9918) -> (43.2354, 53.7952)
  line L294 (37.9212, 51.766) -> (37.9212, 53.0614)
  line L295 (43.2354, 53.7952) -> (43.6369, 57.6889)
  line L296 (30.8262, 49.4754) -> (30.8262, 52.9129)
  line L297 (45.2285, 57.5248) -> (45.3919, 59.1098)
  line L298 (30.8262, 52.9129) -> (30.8262, 53.9269)
  line L299 (29.2262, 48.1845) -> (29.2262, 52.9038)
  line L300 (45.0116, 63.8871) -> (49.5335, 59.4079)
  line L301 (32.0809, 42.0059) -> (30.545, 46.3953)
  line L302 (35.4701, 54.4615) -> (36.6553, 54.1781)
  line L303 (67.0915, 76.678) -> (73.3235, 75.4057)
  line L304 (67.5013, 84.1835) -> (72.3151, 82.9469)
  line L305 (73.8681, 84.1998) -> (72.3108, 89.4858)
  line L306 (81.5527, 88.0664) -> (81.4267, 88.284)
  line L307 (75.2158, 85.2871) -> (73.8403, 89.9558)
  line L308 (76.1584, 84.0186) -> (82.6775, 81.2002)
  line L309 (74.9383, 82.4259) -> (74.7548, 82.8823)
  line L310 (68.3889, 83.9555) -> (72.2959, 82.9518)
  line L311 (79.314, 96.6555) -> (78.9776, 97.5027)
  line L312 (74.7548, 82.8823) -> (82.0425, 79.7315)
  line L313 (73.6436, 76.9733) -> (75.564, 76.5813)
  line L314 (79.6597, 89.856) -> (80.4342, 89.497)
  line L315 (68.7023, 77.9821) -> (73.6436, 76.9733)
  line L316 (68.7436, 85.5164) -> (72.6899, 84.5025)
  line L317 (91.2777, 84.7783) -> (92.4617, 84.1384)
  line L318 (45.3919, 59.1098) -> (49.5335, 59.4079)
  line L319 (36.7393, 55.6397) -> (36.8736, 57.9769)
  line L320 (31.8569, 48.1516) -> (35.5924, 47.0141)
  line L321 (32.3111, 53.5718) -> (35.0977, 52.9055)
  line L322 (32.6725, 55.1305) -> (35.4701, 54.4615)
  line L323 (39.5819, 54.4059) -> (42.0597, 53.9918)
  line L324 (40.7069, 60.6805) -> (42.7105, 60.6319)
  line L325 (22.1293, 42.4591) -> (21.2525, 48.0608)
  line L326 (16.6491, 44.0078) -> (24.5394, 36.1175)
  line L327 (22.7358, 48.9312) -> (27.7829, 47.0202)
  line L328 (24.5394, 36.1175) -> (26.1093, 34.5476)
  line L329 (23.5672, 43.6191) -> (22.7358, 48.9312)
  line L330 (21.9883, 43.3599) -> (21.2525, 48.0608)
  line L331 (29.2262, 49.4693) -> (29.2262, 52.9129)
  line L332 (46.392, 62.0332) -> (46.4462, 62.4661)
  line L333 (42.7105, 60.6319) -> (44.5984, 60.5862)
  line L334 (35.5924, 47.0141) -> (36.3212, 46.7922)
  line L335 (45.0146, 55.4505) -> (45.2285, 57.5248)
  line L336 (37.9212, 53.0614) -> (41.7959, 52.4137)
  line L337 (15.7266, 44.9303) -> (22.1293, 42.4591)
  line L338 (21.0824, 39.4285) -> (91.6554, 96.5652)
  line L339 (-15.7266, 44.9303) -> (-22.1293, 42.4591)
  line L340 (19.9851, 40.7292) -> (90.7737, 97.8385)
  line L341 (-19.9851, 40.7292) -> (-90.7737, 97.8385)
  spline S7 degree 5 poles (-89.5561, 115.7344) (-88.3548, 113.9314) (-85.9183, 110.3595) (-82.1609, 105.1037) (-76.9426, 98.3036) (-70.0489, 90.1727) (-62.7516, 82.4437) (-55.0184, 75.1487) (-46.833, 68.3041) (-38.2146, 61.8908) (-29.1964, 55.8754) (-21.6887, 51.3552) (-15.9034, 48.1188) (-11.9791, 46.0284) (-10, 45) knots -1 -1 -1 -1 -1 -1 -0.9 -0.8 -0.7 -0.6 -0.5 -0.4 -0.3 -0.2 -0.1 0 0 0 0 0 0
  spline S8 degree 5 poles (-25, 30) (-26.2769, 31.7834) (-28.8813, 35.2989) (-32.9395, 40.4185) (-38.6588, 46.9323) (-46.356, 54.5193) (-54.6474, 61.5042) (-63.577, 67.8424) (-73.161, 73.5176) (-83.3647, 78.5649) (-92.6931, 82.436) (-100.1552, 85.1208) (-105.5101, 86.8635) (-108.6093, 87.8146) (-109.3801, 88.0477) knots 0 0 0 0 0 0 0.1 0.2 0.3 0.4 0.5 0.6 0.7 0.8 0.9 0.932954 0.932954 0.932954 0.932954 0.932954 0.932954
  arc A15 (-109.3801, 88.0477) -> (-89.5561, 115.7344) centre (-108, 108) ccw
  line L342 (-45.3919, 59.1098) -> (-49.5335, 59.4079)
  line L343 (-75.564, 76.5813) -> (-73.4538, 81.829)
  line L344 (-60.0386, 76.6835) -> (-64.4078, 76.5676)
  line L345 (-53.3931, 70.682) -> (-58.101, 66.0186)
  line L346 (-66.3286, 78.1172) -> (-66.0088, 82.615)
  line L347 (-63.7187, 71.3413) -> (-66.0187, 71.228)
  line L348 (-101.5784, 88.6355) -> (-102.9173, 87.9717)
  line L349 (-36.3212, 46.7922) -> (-36.3212, 51.766)
  line L350 (-64.4987, 76.5652) -> (-65.6021, 75.4722)
  line L351 (-45.2285, 57.5248) -> (-45.3919, 59.1098)
  line L352 (-29.2262, 49.4693) -> (-29.2262, 52.9129)
  line L353 (-31.8569, 48.1516) -> (-35.5924, 47.0141)
  line L354 (-53.3931, 70.682) -> (-57.6141, 71.0867)
  line L355 (-58.101, 66.0186) -> (-58.8192, 69.9806)
  line L356 (-67.5366, 72.1422) -> (-67.1945, 75.6285)
  line L357 (-76.1584, 84.0186) -> (-82.6775, 81.2002)
  line L358 (-68.7023, 77.9821) -> (-73.6436, 76.9733)
  line L359 (-73.5557, 90.9221) -> (-79.0459, 88.377)
  line L360 (-35.4701, 54.4615) -> (-36.6553, 54.1781)
  line L361 (-57.6141, 71.0867) -> (-58.1695, 74.9342)
  line L362 (-38.3359, 55.5339) -> (-38.471, 57.8848)
  line L363 (-64.4912, 78.166) -> (-66.3286, 78.1172)
  line L364 (-24.5394, 36.1175) -> (-26.1093, 34.5476)
  line L365 (-30.224, 40.7724) -> (-30.8842, 40.5813)
  line L366 (-76.996, 77.3086) -> (-74.9383, 82.4259)
  line L367 (-74.7548, 82.8823) -> (-82.0425, 79.7315)
  line L368 (-81.7381, 90.5489) -> (-79.314, 96.6555)
  line L369 (-38.5427, 59.1325) -> (-42.6724, 59.0324)
  line L370 (-61.6594, 78.2411) -> (-64.4912, 78.166)
  line L371 (-67.0915, 76.678) -> (-73.3235, 75.4057)
  line L372 (-73.6436, 76.9733) -> (-75.564, 76.5813)
  line L373 (-27.8043, 47.0121) -> (-29.0347, 45.8668)
  line L374 (-67.1945, 75.6285) -> (-67.0915, 76.678)
  line L375 (-67.5013, 84.1835) -> (-72.3151, 82.9469)
  line L376 (-57.8815, 72.939) -> (-58.1478, 74.7839)
  line L377 (-67.6012, 82.7793) -> (-67.5013, 84.1835)
  line L378 (-66.0187, 71.228) -> (-65.6021, 75.4722)
  line L379 (-60.6844, 71.4907) -> (-63.7187, 71.3413)
  line L380 (-42.0597, 53.9918) -> (-43.2354, 53.7952)
  line L381 (-93.7857, 85.0368) -> (-87.9816, 93.5909)
  line L382 (-22.1293, 42.4591) -> (-21.2525, 48.0608)
  line L383 (-59.4437, 72.5628) -> (-59.7672, 74.8031)
  line L384 (-73.975, 90.7277) -> (-78.9919, 88.4021)
  line L385 (-86.4629, 107.5181) -> (-88.083, 109.8203)
  line L386 (-59.7672, 74.8031) -> (-60.0386, 76.6835)
  line L387 (-89.3497, 94.6985) -> (-101.5784, 88.6355)
  line L388 (-35.5924, 47.0141) -> (-36.3212, 46.7922)
  line L389 (-45.0146, 55.4505) -> (-45.2285, 57.5248)
  line L390 (-91.2777, 84.7783) -> (-92.4617, 84.1384)
  line L391 (-32.3111, 53.5718) -> (-35.0977, 52.9055)
  line L392 (-72.6899, 84.5025) -> (-73.8681, 84.1998)
  line L393 (-47.5667, 60.8705) -> (-48.0238, 60.9034)
  line L394 (-79.6597, 89.856) -> (-80.4342, 89.497)
  line L395 (-73.8403, 89.9558) -> (-73.5557, 90.9221)
  line L396 (-68.7436, 85.5164) -> (-72.6899, 84.5025)
  line L397 (-36.7393, 55.6397) -> (-36.8736, 57.9769)
  line L398 (-46.392, 62.0332) -> (-46.4462, 62.4661)
  line L399 (-67.8456, 79.3411) -> (-67.6012, 82.7793)
  line L400 (-85.3974, 81.4245) -> (-81.5527, 88.0664)
  line L401 (-73.6551, 84.9229) -> (-72.3584, 89.3243)
  line L402 (-58.8192, 69.9806) -> (-63.64, 69.7432)
  line L403 (-80.2171, 90.0439) -> (-77.908, 95.8607)
  line L404 (-23.9305, 48.4789) -> (-27.8043, 47.0121)
  line L405 (-79.314, 96.6555) -> (-78.9776, 97.5027)
  line L406 (-75.2158, 85.2871) -> (-73.8403, 89.9558)
  line L407 (-40.7069, 60.6805) -> (-42.7105, 60.6319)
  line L408 (-87.9816, 93.5909) -> (-100.8677, 87.202)
  line L409 (-80.4342, 89.497) -> (-77.8281, 96.0622)
  line L410 (-32.6725, 55.1305) -> (-35.4701, 54.4615)
  line L411 (-66.2418, 79.3387) -> (-66.006, 82.6541)
  line L412 (-37.9212, 48.4975) -> (-37.9212, 51.766)
  line L413 (-28.3781, 48.5056) -> (-29.2262, 48.1845)
  line L414 (-74.6324, 92.1865) -> (-79.6597, 89.856)
  line L415 (-37.9212, 53.0614) -> (-41.7959, 52.4137)
  line L416 (-36.6553, 54.1781) -> (-36.873, 57.9658)
  line L417 (-81.4267, 88.284) -> (-90.517, 83.3708)
  line L418 (-37.9212, 51.766) -> (-37.9212, 53.0614)
  line L419 (-23.5672, 43.6191) -> (-22.7358, 48.9312)
  line L420 (-68.3889, 83.9555) -> (-72.2959, 82.9518)
  line L421 (-21.9883, 43.3599) -> (-21.2525, 48.0608)
  line L422 (-85.3974, 81.4245) -> (-85.4862, 81.271)
  line L423 (-42.7105, 60.6319) -> (-44.5984, 60.5862)
  line L424 (-73.8681, 84.1998) -> (-72.3108, 89.4858)
  line L425 (-93.7857, 85.0368) -> (-93.9955, 84.7275)
  line L426 (-24.7124, 42.3674) -> (-30.224, 40.7724)
  line L427 (-74.9383, 82.4259) -> (-74.7548, 82.8823)
  line L428 (-86.334, 95.1053) -> (-86.9472, 94.7515)
  line L429 (-81.5527, 88.0664) -> (-81.4267, 88.284)
  line L430 (-82.6775, 81.2002) -> (-84.0126, 80.6229)
  line L431 (-101.1598, 87.3016) -> (-104.0335, 88.3973)
  line L432 (-92.4617, 84.1384) -> (-86.7336, 92.5805)
  line L433 (-43.2354, 53.7952) -> (-43.6369, 57.6889)
  line L434 (-30.545, 46.3953) -> (-30.3557, 46.9362)
  line L435 (-16.6491, 44.0078) -> (-24.5394, 36.1175)
  line L436 (-44.5984, 60.5862) -> (-45.0116, 63.8871)
  line L437 (-24.4898, 49.9779) -> (-28.3781, 48.5056)
  line L438 (-30.8262, 52.9129) -> (-30.8262, 53.9269)
  line L439 (-39.5819, 54.4059) -> (-42.0597, 53.9918)
  line L440 (-38.471, 57.8848) -> (-38.5427, 59.1325)
  line L441 (-82.7739, 89.3746) -> (-91.2777, 84.7783)
  line L442 (-45.0116, 63.8871) -> (-49.5335, 59.4079)
  line L443 (-22.7358, 48.9312) -> (-27.7829, 47.0202)
  line L444 (-18.5197, 42.1372) -> (-20.6913, 41.299)
  line L445 (82.7739, 89.3746) -> (91.2777, 84.7783)
  line L446 (87.9816, 93.5909) -> (100.8677, 87.202)
  line L447 (85.3974, 81.4245) -> (81.5527, 88.0664)
  line L448 (82.6775, 81.2002) -> (84.0126, 80.6229)
  line L449 (101.1598, 87.3016) -> (104.0335, 88.3973)
  line L450 (93.7857, 85.0368) -> (87.9816, 93.5909)
  line L451 (84.0126, 80.6229) -> (80.1679, 87.2648)
  line L452 (79.1831, 97.3842) -> (85.5398, 93.7163)
  line L453 (81.4267, 88.284) -> (90.517, 83.3708)
  line L454 (78.9776, 97.5027) -> (85.6123, 93.6745)
  line L455 (79.9758, 98.774) -> (86.334, 95.1053)
  line L456 (-22.1293, 42.4591) -> (-23.1969, 41.1404)
  line L457 (-29.2262, 48.1845) -> (-29.2262, 52.9038)
  line L458 (-23.1969, 41.1404) -> (-26.1093, 34.5476)
  spline S9 degree 3 poles (26.1093, 34.5476) (33.7424, 44.66) (42.377, 53.7768) (52.2721, 61.6437) (60.5587, 68.2317) (69.767, 73.8901) (79.7914, 78.6767) (86.5715, 81.9141) (93.7109, 84.7689) (101.1598, 87.3016) knots 0.039267 0.039267 0.039267 0.039267 0.383484 0.383484 0.383484 0.671746 0.671746 0.671746 0.86671 0.86671 0.86671 0.86671
  spline S10 degree 3 poles (86.4629, 107.5181) (77.6632, 95.0692) (67.8257, 83.6168) (56.6007, 73.5039) (44.7534, 62.8301) (31.3991, 53.6699) (16.9588, 45.6135) (16.549, 45.3849) (16.1382, 45.1571) (15.7266, 44.9303) knots -0.921557 -0.921557 -0.921557 -0.921557 -0.5 -0.5 -0.5 -0.055069 -0.055069 -0.055069 -0.042441 -0.042441 -0.042441 -0.042441
  line L459 (-21.9085, 40.0973) -> (-22.9759, 37.6809)
  spline S11 degree 5 poles (89.5561, 115.7344) (88.3548, 113.9314) (85.9183, 110.3595) (82.1609, 105.1037) (76.9426, 98.3036) (70.0489, 90.1727) (62.7516, 82.4437) (55.0184, 75.1487) (46.833, 68.3041) (38.2146, 61.8908) (29.1964, 55.8754) (21.6887, 51.3552) (15.9034, 48.1188) (11.9791, 46.0284) (10, 45) knots -1 -1 -1 -1 -1 -1 -0.9 -0.8 -0.7 -0.6 -0.5 -0.4 -0.3 -0.2 -0.1 0 0 0 0 0 0
  line L460 (-23.1969, 41.1404) -> (-29.7792, 39.2354)
  line L461 (-30.8262, 49.4754) -> (-30.8262, 52.9129)
  line L462 (-16.6491, 44.0078) -> (-15.7266, 44.9303)
  line L463 (-30.8842, 40.5813) -> (-29.0347, 45.8668)
  line L464 (-21.0824, 39.4285) -> (-91.6554, 96.5652)
  spline S12 degree 3 poles (-86.4629, 107.5181) (-77.6632, 95.0692) (-67.8257, 83.6168) (-56.6007, 73.5039) (-44.7534, 62.8301) (-31.3991, 53.6699) (-16.9588, 45.6135) (-16.549, 45.3849) (-16.1382, 45.1571) (-15.7266, 44.9303) knots -0.921557 -0.921557 -0.921557 -0.921557 -0.5 -0.5 -0.5 -0.055069 -0.055069 -0.055069 -0.042441 -0.042441 -0.042441 -0.042441
  line L465 (-79.1831, 97.3842) -> (-85.5398, 93.7163)
  line L466 (-30.3557, 46.9362) -> (-35.1263, 45.4835)
  line L467 (-84.0126, 80.6229) -> (-80.1679, 87.2648)
  line L468 (-30.8262, 53.9269) -> (-35.0824, 52.9091)
  line L469 (-32.0809, 42.0059) -> (-30.545, 46.3953)
  line L470 (-61.718, 76.639) -> (-64.4987, 76.5652)
  line L471 (-79.9758, 98.774) -> (-86.334, 95.1053)
  line L472 (-78.9776, 97.5027) -> (-85.6123, 93.6745)
  spline S13 degree 3 poles (-26.1093, 34.5476) (-33.7424, 44.66) (-42.377, 53.7768) (-52.2721, 61.6437) (-60.5587, 68.2317) (-69.767, 73.8901) (-79.7914, 78.6767) (-86.5715, 81.9141) (-93.7109, 84.7689) (-101.1598, 87.3016) knots 0.039267 0.039267 0.039267 0.039267 0.383484 0.383484 0.383484 0.671746 0.671746 0.671746 0.86671 0.86671 0.86671 0.86671
  line L473 (66.3286, 78.1172) -> (66.0088, 82.615)
  line L474 (75.564, 76.5813) -> (73.4538, 81.829)
  line L475 (81.7381, 90.5489) -> (79.314, 96.6555)
  line L476 (80.2171, 90.0439) -> (77.908, 95.8607)
  line L477 (74.6324, 92.1865) -> (79.6597, 89.856)
  line L478 (80.4342, 89.497) -> (77.8281, 96.0622)
  line L479 (67.8456, 79.3411) -> (67.6012, 82.7793)
  line L480 (73.975, 90.7277) -> (78.9919, 88.4021)
  line L481 (73.8403, 89.9558) -> (73.5557, 90.9221)
  line L482 (76.996, 77.3086) -> (74.9383, 82.4259)
  line L483 (73.6551, 84.9229) -> (72.3584, 89.3243)
  line L484 (67.6012, 82.7793) -> (67.5013, 84.1835)
  line L485 (73.5557, 90.9221) -> (79.0459, 88.377)
  line L486 (72.6899, 84.5025) -> (73.8681, 84.1998)
  line L487 (92.4617, 84.1384) -> (86.7336, 92.5805)
  line L488 (86.334, 95.1053) -> (86.9472, 94.7515)
  line L489 (93.7857, 85.0368) -> (93.9955, 84.7275)
  line L490 (85.3974, 81.4245) -> (85.4862, 81.271)
  line L491 (101.5784, 88.6355) -> (102.9173, 87.9717)
  line L492 (89.3497, 94.6985) -> (101.5784, 88.6355)
  line L493 (84.24, 103.2596) -> (83.881, 103.9354)
  line L494 (86.4629, 107.5181) -> (88.083, 109.8203)
  arc A16 (89.5561, 115.7344) -> (109.3801, 88.0477) centre (108, 108) ccw
  line L495 (59.7672, 74.8031) -> (60.0386, 76.6835)
  line L496 (58.8192, 69.9806) -> (63.64, 69.7432)
  line L497 (61.6594, 78.2411) -> (64.4912, 78.166)
  line L498 (53.3931, 70.682) -> (58.101, 66.0186)
  line L499 (57.6141, 71.0867) -> (58.1695, 74.9342)
  line L500 (66.2418, 79.3387) -> (66.006, 82.6541)
  line L501 (59.4437, 72.5628) -> (59.7672, 74.8031)
  line L502 (61.718, 76.639) -> (64.4987, 76.5652)
  line L503 (64.4912, 78.166) -> (66.3286, 78.1172)
  line L504 (67.1945, 75.6285) -> (67.0915, 76.678)
  line L505 (-10, 45) -> (-25, 30)
  line L506 (53.3931, 70.682) -> (57.6141, 71.0867)
  line L507 (60.6844, 71.4907) -> (63.7187, 71.3413)
  line L508 (57.8815, 72.939) -> (58.1478, 74.7839)
  line L509 (63.7187, 71.3413) -> (66.0187, 71.228)
  line L510 (67.5366, 72.1422) -> (67.1945, 75.6285)
  line L511 (66.0187, 71.228) -> (65.6021, 75.4722)
  line L512 (60.0386, 76.6835) -> (64.4078, 76.5676)
  line L513 (64.4987, 76.5652) -> (65.6021, 75.4722)
  line L514 (58.101, 66.0186) -> (58.8192, 69.9806)
  line L515 (-10, -45) -> (10, -45)
  spline S14 degree 5 poles (10, -45) (11.9791, -46.0284) (15.9034, -48.1188) (21.6887, -51.3552) (29.1964, -55.8754) (38.2146, -61.8908) (46.833, -68.3041) (55.0184, -75.1487) (62.7516, -82.4437) (70.0489, -90.1727) (76.9426, -98.3036) (82.1609, -105.1037) (85.9183, -110.3595) (88.3548, -113.9314) (89.5561, -115.7344) knots 0 0 0 0 0 0 0.1 0.2 0.3 0.4 0.5 0.6 0.7 0.8 0.9 1 1 1 1 1 1
  arc A17 (109.3801, -88.0477) -> (89.5561, -115.7344) centre (108, -108) ccw
  spline S15 degree 5 poles (109.3801, -88.0477) (108.6093, -87.8146) (105.5101, -86.8635) (100.1552, -85.1208) (92.6931, -82.436) (83.3647, -78.5649) (73.161, -73.5176) (63.577, -67.8424) (54.6474, -61.5042) (46.356, -54.5193) (38.6588, -46.9323) (32.9395, -40.4185) (28.8813, -35.2989) (26.2769, -31.7834) (25, -30) knots -0.932954 -0.932954 -0.932954 -0.932954 -0.932954 -0.932954 -0.9 -0.8 -0.7 -0.6 -0.5 -0.4 -0.3 -0.2 -0.1 0 0 0 0 0 0
  line L516 (25, -30) -> (25, 30)
  spline S16 degree 5 poles (25, 30) (26.2769, 31.7834) (28.8813, 35.2989) (32.9395, 40.4185) (38.6588, 46.9323) (46.356, 54.5193) (54.6474, 61.5042) (63.577, 67.8424) (73.161, 73.5176) (83.3647, 78.5649) (92.6931, 82.436) (100.1552, 85.1208) (105.5101, 86.8635) (108.6093, 87.8146) (109.3801, 88.0477) knots 0 0 0 0 0 0 0.1 0.2 0.3 0.4 0.5 0.6 0.7 0.8 0.9 0.932954 0.932954 0.932954 0.932954 0.932954 0.932954
  arc A18 (89.5561, 115.7344) -> (109.3801, 88.0477) centre (108, 108) ccw
  spline S17 degree 5 poles (89.5561, 115.7344) (88.3548, 113.9314) (85.9183, 110.3595) (82.1609, 105.1037) (76.9426, 98.3036) (70.0489, 90.1727) (62.7516, 82.4437) (55.0184, 75.1487) (46.833, 68.3041) (38.2146, 61.8908) (29.1964, 55.8754) (21.6887, 51.3552) (15.9034, 48.1188) (11.9791, 46.0284) (10, 45) knots -1 -1 -1 -1 -1 -1 -0.9 -0.8 -0.7 -0.6 -0.5 -0.4 -0.3 -0.2 -0.1 0 0 0 0 0 0
  line L517 (10, 45) -> (-10, 45)